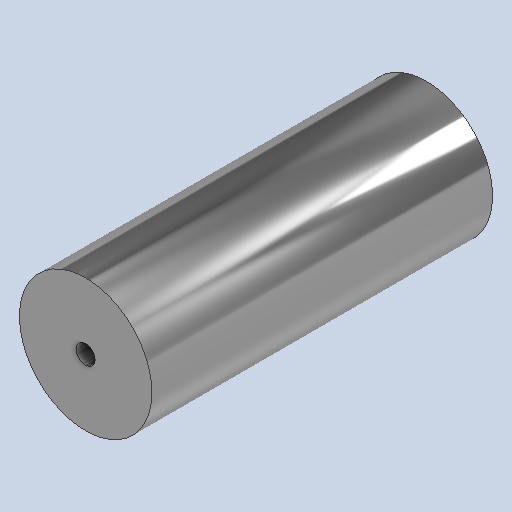
# Autodesk Inventor part: Part9
Saved by Autodesk Inventor 2022.3 (Build 263350000, 350)
## iProperties
Created: 2022-11-16
Part Number: Part9
Material: Silicon Nitride
Document SubType Name: Modeling
Designer: komputer
Mass: 106.576 g
Surface Area: 96.9894 cm^2
Volume: 33.5144 cm^3
Density: 3.18 g/cm^3
Appearance: Chrome - Polished Black
Author: komputer
Autodesk Inventor part; units mm, degrees
ref_plane "YZ Plane" through (0, 0, 0) normal (1, 0, 0) x (0, 1, 0)
ref_plane "XZ Plane" through (0, 0, 0) normal (0, 1, 0) x (-1, 0, 0)
ref_plane "XY Plane" through (0, 0, 0) normal (0, 0, 1) x (1, 0, 0)
sketch "Sketch1" plane through (0, 0, 0) normal (0, 0, 1) x (1, 0, 0)
  line L0 (-1.118, -1.25) -> (1.118, -1.25) projected
  arc A0 (1.118, -1.25) -> (-1.118, -1.25) centre (0, -0.25) ccw projected
  circle A1 centre (-0.0155, -0.3768) radius 13 projected
  line L1 (7.9845, 2.6232) -> (7.9845, -0.3768) projected
  arc A2 (3.9845, -7.3768) -> (7.9845, -3.3768) centre (3.9845, -3.3768) ccw projected
  line L2 (3.9845, -7.3768) -> (-4.0155, -7.3768) projected
  arc A3 (-8.0155, -3.3768) -> (-4.0155, -7.3768) centre (-4.0155, -3.3768) ccw projected
  line L3 (-8.0155, -3.3768) -> (-8.0155, 2.6232) projected
  arc A4 (-6.0155, 6.0873) -> (-8.0155, 2.6232) centre (-4.0155, 2.6232) ccw projected
  line L4 (-6.0155, 6.0873) -> (-6.0155, -0.3768) projected
  arc A5 (-6.0155, -0.3768) -> (-3.3321, -5.3768) centre (-0.0155, -0.3768) ccw projected
  line L5 (-3.3321, -5.3768) -> (3.3011, -5.3768) projected
  arc A6 (3.3011, -5.3768) -> (5.9845, -0.3768) centre (-0.0155, -0.3768) ccw projected
  line L6 (5.9845, -0.3768) -> (5.9845, 6.0873) projected
  arc A7 (7.9845, 2.6232) -> (5.9845, 6.0873) centre (3.9845, 2.6232) ccw projected
  circle A8 centre (0, 0) radius 11
  line L7 (0, 11) -> (0, 14)
  circle A9 centre (0, 0) radius 14
  circle A10 centre (9.4845, -0.3768) radius 1.5 projected
  line L8 (7.9845, -0.3768) -> (7.9845, -3.3768) projected
  dimension "d0" = 22
  dimension "d1" = 3
  constraints: 2 coincident, 2 end point, 2 vertical alignment, 1 horizontal alignment, 1 vertical, 4 other
  measures "d1" distance of L7.start L7.end
extrude "Extrusion1" add sketch "Sketch1" against normal blind 8 contours A8 | A1 | A9 | A10 | L1 L8 A2 L2 A3 L3 A4 L4 A5 L5 A6 L6 A7
sketch "Sketch2" plane through (0, 0, -8) normal (0, 0, -1) x (-1, 0, 0)
  circle A0 centre (0, 0) radius 14 projected
  arc A1 (1.118, -1.25) -> (-1.118, -1.25) centre (0, -0.25) ccw projected
  line L0 (1.118, -1.25) -> (-1.118, -1.25) projected
  circle A2 centre (0, 0) radius 14 projected
  line L1 (-14, 0) -> (-11, 0)
  circle A3 centre (0, 0) radius 11
  dimension "d4" = 3
  constraints: 2 end point, 2 horizontal alignment, 1 coincident, 1 horizontal, 3 other
  measures "d4" distance of L1.start L1.end
extrude "Extrusion2" add sketch "Sketch2" along normal blind 28 contours A0
sketch "Sketch3" plane through (0, 0, 0) normal (0, 0, 1) x (1, 0, 0)
  circle A0 centre (0, 0) radius 14 projected
extrude "Extrusion3" add sketch "Sketch3" along normal blind 36
sketch "Sketch4" plane through (0, 0, 36) normal (0, 0, 1) x (1, 0, 0)
  circle A0 centre (0, 0) radius 2 projected
  point P0 (0, 0)
extrude "Extrusion4" cut sketch "Sketch4" against normal blind 10
body "Solid1"
